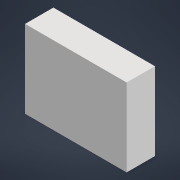
# Autodesk Inventor part: FakeV
Saved by Autodesk Inventor 2022 (Build 260153070, 153G)
## iProperties
Created: 2021-12-13
Part Number: FakeV
Material: Типовые
Document SubType Name: Modeling
Designer: kalugin_a
Density: 1 g/cm^3
Appearance: По умолчанию
Author: kalugin_a
Autodesk Inventor part; units mm, degrees
ref_plane "YZ Plane" through (0, 0, 0) normal (1, 0, 0) x (0, 1, 0)
ref_plane "XZ Plane" through (0, 0, 0) normal (0, 1, 0) x (-1, 0, 0)
ref_plane "XY Plane" through (0, 0, 0) normal (0, 0, 1) x (1, 0, 0)
sketch "Эскиз1" plane through (0, 0, 0) normal (0, 0, 1) x (1, 0, 0)
  line L0 (0, 0) -> (218, 0)
  line L1 (218, 0) -> (218, 162)
  line L2 (218, 162) -> (0, 162)
  line L3 (0, 162) -> (0, 0)
  dimension "d0" = 218
  dimension "d1" = 162
  constraints: 8 end point, 2 parallel, 1 horizontal, 1 perpendicular
  measures "d0" distance of L2.end L1.end
  measures "d1" distance of L1.end L0.end
extrude "Выдавливание1" add sketch "Эскиз1" along normal blind 61
